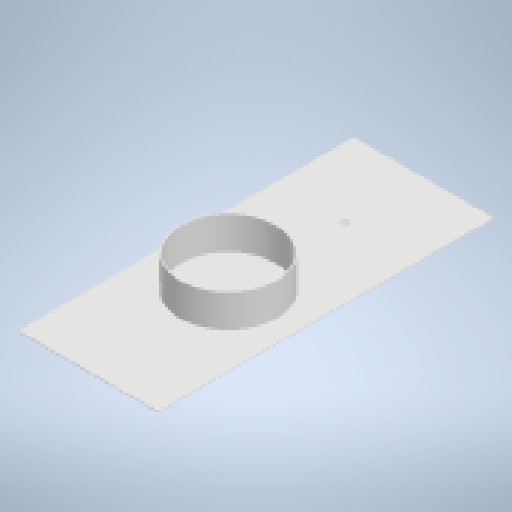
# Autodesk Inventor part: mid Base
Saved by Autodesk Inventor 2025.2 (Build 292293000, 293)
## iProperties
Created: 2025-05-26
Part Number: mid Base
Material: Generic
Document SubType Name: Sheet Metal
Designer: abdal
Density: 1 g/cm^3
Sheet Metal Rule: Default_mm
Appearance: Default
Author: abdal
Autodesk Inventor part; units mm, degrees
ref_plane "YZ Plane" through (0, 0, 0) normal (1, 0, 0) x (0, 1, 0)
ref_plane "XZ Plane" through (0, 0, 0) normal (0, 1, 0) x (-1, 0, 0)
ref_plane "XY Plane" through (0, 0, 0) normal (0, 0, 1) x (1, 0, 0)
sketch "Sketch1" plane through (0, 0, 0) normal (0, 1, 0) x (-1, 0, 0)
  line L0 (215, 515) -> (-215, 515)
  line L1 (-215, 515) -> (-215, -515)
  line L2 (-215, -515) -> (215, -515)
  line L3 (215, -515) -> (215, 515)
  line L4 (215, 515) -> (-215, -515) construction
  line L5 (-215, 515) -> (215, -515) construction
  point P0 (0, 0)
  dimension "d0" = 430
  dimension "d1" = 1030
  measures "d0" distance of L1.end L2.end
  measures "d1" distance of L2.end L0.start
extrude "Plate1" add sketch "Sketch1" along normal blind 2
sketch "Sketch2" plane through (0, 2, 0) normal (0, 1, 0) x (1, 0, 0)
  circle A0 centre (0, -85) radius 145
  line L0 (215, -515) -> (-215, -515) projected
  circle A1 centre (0, -85) radius 149
  point P0 (0, 0)
  dimension "d3" = 430
  dimension "d4" = 290
  dimension "d5" = 0
  dimension "d6" = 4
  constraints: 2 centre point
  measures "d3" distance from line of L0 A0.centre
  measures "d4" diameter of A0
  measures "d5" horizontal distance of point (0, 0) A0.centre
  measures "d6" radial gap between concentric circles of A0 A1
extrude "Extrusion1" add sketch "Sketch2" along normal blind 100
sketch "Sketch3" plane through (0, 2, 0) normal (0, 1, 0) x (1, 0, 0)
  circle A0 centre (0, 273.2302) radius 10.795
  point P0 (0, 0)
  dimension "d10" = 21.59
  constraints: 1 centre point
  measures "d10" diameter of A0
extrude "Cut1" cut sketch "Sketch3" against normal through all
equation "\"d11\" = Thickness"
equation "\"d2\" = Thickness"
equation "\"BendRadius\" = Thickness"
equation "\"BendReliefWidth\" = Thickness"
equation "\"BendReliefDepth\" = 0.5 * Thickness"
equation "\"CornerReliefSize\" = 4 * Thickness"
equation "\"MinimumRemnant\" = 2 * Thickness"
equation "\"TransitionRadius\" = BendRadius"
equation "\"JacobiRadiusSize\" = BendRadius"
equation "\"GapSize\" = Thickness"
equation "\"Thickness\" = 2"
body "Solid1"
